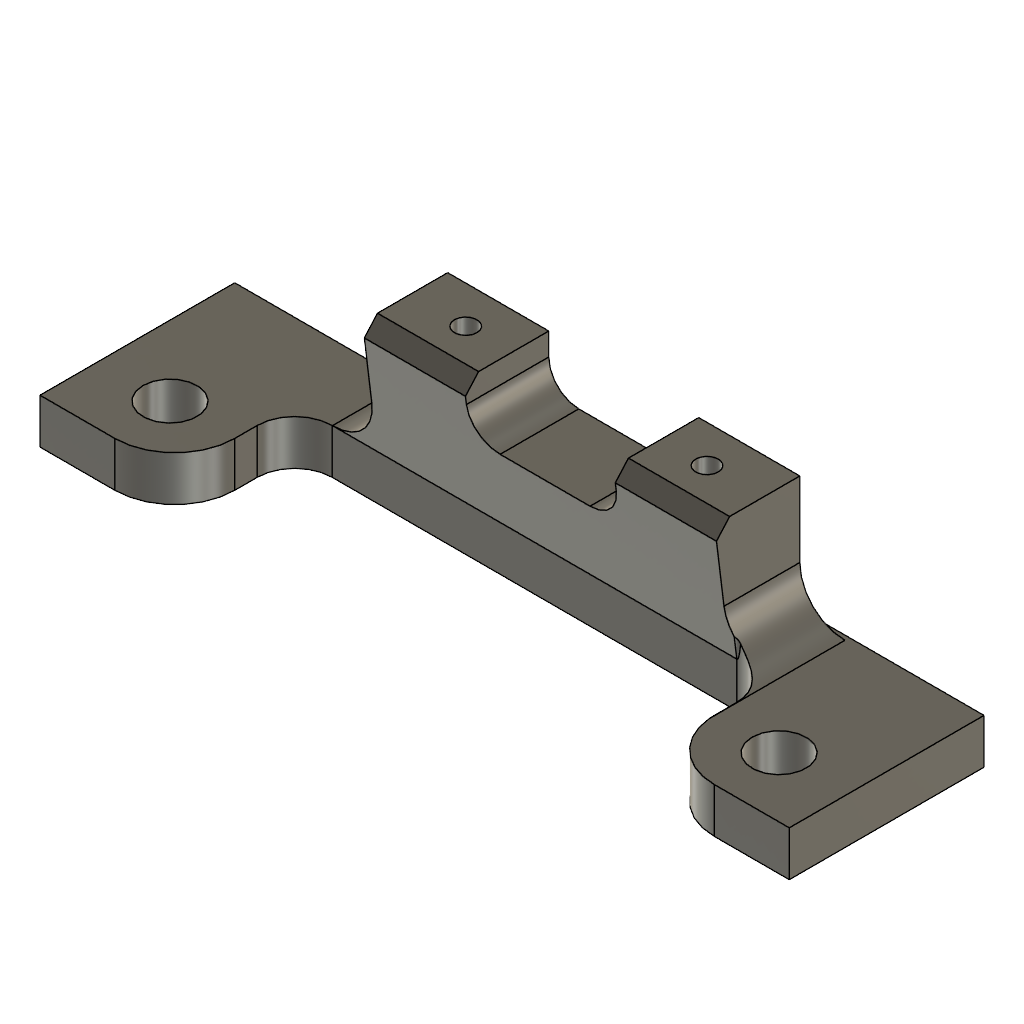
Traeger (Autodesk Fusion 360 design; units mm, degrees)
Autodesk Fusion 360 part; units mm, degrees
sketch "Skizze1" plane through (0, 0, 0) normal (0, 0, 1) x (1, 0, 0)
  line L0 (0, 0) -> (-50, 0)
  line L1 (-50, 0) -> (-50, 13)
  line L2 (-50, 13) -> (0, 13)
  line L3 (0, 13) -> (0, 0)
  circle A0 centre (-4.68, 4) radius 1.8
  circle A1 centre (-45.32, 4) radius 1.8
  line L4 (-50, 4) -> (0, 4) construction
  line L5 (-25, 13) -> (-25, 0) construction
  line L6 (-41, 0) -> (-41, 8)
  line L7 (-41, 8) -> (-9, 8)
  line L8 (-9, 8) -> (-9, 0)
  dimension "d1" = 50
  dimension "d2" = 13
  dimension "d3" = 3.6
  dimension "d4" = 40.64
  dimension "d5" = 9
  dimension "d11" = 5
  dimension "d12" = 9
  dimension "d13" = 9
  constraint horizontal L0
  constraint vertical L1
  constraint horizontal L2
  constraint vertical L3
  constraint coincident L0.start L3.end
  constraint coincident L1 L4.start
  constraint coincident L3 L4.end
  constraint perpendicular L3 L4
  constraint coincident A1.centre L4
  constraint coincident A0.centre L4
  constraint equal A0 A1
  constraint midpoint L2 L5.start
  constraint midpoint L0 L5.end
  constraint symmetric A0.centre A1.centre L5
  constraint coincident L0 L6.start
  constraint perpendicular L4 L6
  constraint perpendicular L6 L7
  constraint coincident L0 L8.end
  constraint perpendicular L0 L8
  measures "d1" distance of L0.start L0.end
  measures "d2" distance of L0.end L1.end
  measures "d3" diameter of A1
  measures "d4" distance of A0.centre A1.centre
  measures "d5" distance of L2 L4
  measures "d11" distance of L2 L7
  measures "d12" distance of L1 L6
  measures "d13" distance of L3 L8
extrude "Extrusion1" add sketch "Skizze1" along normal blind 3 contours L0 L1 L2 L3 L6 L7 L8
sketch "Skizze2" plane through (0, 0, 3) normal (0, 0, 1) x (-1, 0, 0)
  circle A0 centre (4.68, -4) radius 1.8
  circle A1 centre (45.32, -4) radius 1.8
  line L0 (41, 0) -> (41, -8)
  line L1 (41, -8) -> (9, -8)
  line L2 (9, 0) -> (0, 0)
  line L3 (0, 0) -> (0, -13)
  line L4 (0, -13) -> (50, -13)
  line L5 (50, -13) -> (50, 0)
  line L6 (50, 0) -> (41, 0)
  line L7 (34.48, -0.19) -> (12.98, -0.19) construction
  line L8 (12.98, -0.19) -> (12.98, -12.69) construction
  line L9 (12.98, -12.69) -> (34.48, -12.69) construction
  line L10 (34.48, -12.69) -> (34.48, -0.19) construction
  circle A2 centre (31.78, -10.19) radius 0.75
  circle A3 centre (15.68, -10.19) radius 0.75
  line L11 (34.48, -10.19) -> (12.98, -10.19) construction
  line L12 (31.78, -12.69) -> (31.78, -0.19) construction
  line L13 (15.68, -12.69) -> (15.68, -0.19) construction
  line L14 (34.48, -1.46) -> (12.98, -1.46) construction
  line L15 (23.73, -12.69) -> (23.73, -0.19) construction
  line L16 (35.48, -8) -> (35.48, -13)
  line L17 (11.98, -8) -> (11.98, -13)
  line L18 (11.98, -12.69) -> (35.48, -12.69)
  point P0 (30.08, -1.46)
  point P1 (17.38, -1.46)
  dimension "d20" = 1.5
  dimension "d21" = 1.5
  dimension "d22" = 21.5
  dimension "d23" = 12.5
  dimension "d25" = 2.5
  dimension "d27" = 1.27
  dimension "d28" = 12.7
  dimension "d29" = 15.24
  dimension "d30" = 12.7
  dimension "d31" = 2.54
  dimension "d32" = 1
  dimension "d33" = 1
  dimension "d51" = 16.1
  constraint horizontal L7
  constraint vertical L8
  constraint horizontal L9
  constraint vertical L10
  constraint coincident L10 L11.start
  constraint coincident L8 L11.end
  constraint perpendicular L8 L11
  constraint coincident L9 L12.start
  constraint coincident L7 L12.end
  constraint perpendicular L7 L12
  constraint coincident L9 L13.start
  constraint coincident L7 L13.end
  constraint perpendicular L7 L13
  constraint coincident A2.centre L11
  constraint coincident A2.centre L12
  constraint coincident A3.centre L13
  constraint coincident A3.centre L11
  constraint coincident L10 L14.start
  constraint coincident L8 L14.end
  constraint perpendicular L8 L14
  constraint coincident L14 P0
  constraint coincident L14 P1
  constraint midpoint L9 L15.start
  constraint midpoint L7 L15.end
  constraint symmetric P0 P1 L15
  constraint coincident L1 L16.start
  constraint coincident L4 L16.end
  constraint coincident L1 L17.start
  constraint coincident L4 L17.end
  constraint vertical L17
  constraint vertical L16
  constraint coincident L17 L18.start
  constraint coincident L16 L18.end
  constraint perpendicular L16 L18
  constraint coincident L8.end L18
  constraint symmetric A2.centre A3.centre L15
  measures "d20" diameter of A2
  measures "d21" diameter of A3
  measures "d22" distance of L7.start L7.end
  measures "d23" distance of L7.start L9.end
  measures "d25" distance of L9 L11
  measures "d27" distance of L7 L14
  measures "d28" distance of P0 P1
  measures "d29" horizontal distance of A1.centre P0
  measures "d30" horizontal distance of A0.centre P1
  measures "d31" vertical distance of A1.centre P0
  measures "d32" distance of L8 L17
  measures "d33" distance of L10 L16
  measures "d51" distance of A2.centre A3.centre
extrude "Extrusion2" add sketch "Skizze2" along normal blind 8 contours L1 L16 L17 L18
sketch "Skizze3" plane through (0, 12.69, 0) normal (0, 1, 0) x (-1, 0, 0)
  line L0 (11.98, 3) -> (35.48, 3)
  line L1 (35.48, 3) -> (35.48, 11)
  line L2 (35.48, 11) -> (11.98, 11)
  line L3 (11.98, 11) -> (11.98, 3)
  line L4 (23.73, 11) -> (23.73, 2.7366) construction
  line L5 (18.73, 7.5) -> (28.73, 7.5)
  line L6 (28.73, 7.5) -> (28.73, 11)
  line L7 (18.73, 7.5) -> (18.73, 11)
  line L8 (18.73, 11) -> (28.73, 11)
  dimension "d37" = 3.5
  dimension "d38" = 10
  constraint midpoint L2 L4.start
  constraint perpendicular L0 L4
  constraint perpendicular L4 L5
  constraint coincident L2 L6.end
  constraint coincident L2 L7.end
  constraint symmetric L4 L6.end L7.end
  constraint symmetric L4 L5.start L5.end
  constraint vertical L7
  measures "d37" distance of L5 L8
  measures "d38" distance of L5.start L5.end
extrude "Extrusion3" cut sketch "Skizze3" against normal up to surface (4.69 mm away) contours L2 L5 L6 L7 L8
fillet "Abrundung1" radius 3 1 edges at (-11.98, 10.345, 3)
fillet "Abrundung2" radius 3 1 edges at (-35.48, 10.345, 3)
fillet "Abrundung3" radius 2 2 edges at (-18.73, 10.345, 7.5) (-28.73, 10.345, 7.5)
fillet "Abrundung4" radius 4 2 edges at (-9, 0, 1.5) (-41, 0, 1.5)
fillet "Abrundung5" radius 2.5 2 edges at (-9, 8, 1.5) (-41, 8, 1.5)
extrude "Extrusion4" add 1 faces at (-25.5767, 8, 2.5) along direction (0, -1, 0) blind 1
sketch "Skizze4" plane through (-38.5, 0, 0) normal (-1, 0, 0) x (0, -1, 0)
  line L0 (-8, 3) -> (-8, 0)
  line L1 (-8, 0) -> (-7, 0)
  line L2 (-7, 0) -> (-7, 3)
  line L3 (-7, 3) -> (-8, 3)
  line L4 (-8, 3) -> (-7, 3)
  line L5 (-7, 11) -> (-12.69, 11)
  line L6 (-12.69, 11) -> (-7, 11)
  line L7 (-10.94, 11) -> (-9.44, 11)
  line L8 (-7, 3) -> (-7, 11)
  line L9 (-8, 3) -> (-7, 11)
  constraint coincident L0.start L3.end
  constraint coincident L2.end L3.start
  constraint coincident L5.start L6.end
extrude "Extrusion5" cut sketch "Skizze4" against normal up to surface (27 mm away)
fillet "Abrundung6" radius 0.3 1 edges at (-11.5, 8, 3.6861)
chamfer "Fase1" distance 1 angle 45 2 edges at (-32.105, 7, 11) (-15.355, 7, 11) tangent chain off
equation "d4 = ( 16 * 2.54 ) * 1 mm"
equation "d13 = d12"
equation "d25 = 1 mm + 1.5 mm"
equation "d27 = ( 2.54 / 2 ) * 1 mm"
equation "d28 = ( 2.54 * 5 ) * 1 mm"
equation "d29 = ( 6 * 2.54 ) * 1 mm"
equation "d34 = 11 mm - 3 mm"
